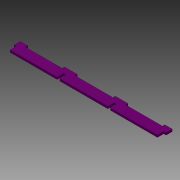
# Autodesk Inventor part: longSlat
Saved by Autodesk Inventor 2015 SP1 (Build 190203100, 203)
## iProperties
Created: 2015-04-09
Part Number: longSlat
Material: Generic
Document SubType Name: Modeling
Designer: Iain
Density: 1 g/cm^3
Appearance: Smooth - Purple
Author: Iain
Autodesk Inventor part; units mm, degrees
ref_plane "YZ Plane" through (0, 0, 0) normal (1, 0, 0) x (0, 1, 0)
sketch "Sketch1" plane through (0, 0, 0) normal (0, 0, 1) x (1, 0, 0)
  line L0 (-590, 40) -> (590, 40)
  line L1 (590, 40) -> (590, -40)
  line L2 (590, -40) -> (-590, -40)
  line L3 (-590, -40) -> (-590, 40)
  point P0 (0, 0)
  point P1 (-590, 0)
  point P2 (0, 40)
  dimension "d0" = 80
  dimension "d1" = 1180
  constraints: 8 end point, 2 midpoint, 2 parallel, 1 horizontal, 1 horizontal alignment, 1 perpendicular, 1 vertical alignment
  measures "d0" distance of L2.end L0.start
  measures "d1" distance of L0.start L0.end
extrude "Extrusion1" add sketch "Sketch1" along normal blind 18
sketch "Sketch2" plane through (0, 0, 18) normal (0, 0, 1) x (1, 0, 0)
  line L0 (590, 40) -> (-590, 40) projected
  line L1 (-590, 40) -> (-590, -40) projected
  line L2 (-590, -40) -> (590, -40) projected
  line L3 (590, -40) -> (590, 40) projected
  line L4 (-590, 58) -> (-531, 58)
  line L5 (-531, 58) -> (-531, 40)
  line L6 (-531, 40) -> (-590, 40)
  line L7 (-590, 40) -> (-590, 58)
  point P0 (0, 0)
  point P1 (-560.5, 40)
  point P2 (0, 40)
  point P3 (-590, 49)
  point P4 (-590, 0)
  dimension "d4" = 18
  dimension "d5" = 59
  constraints: 8 end point, 4 midpoint, 2 parallel, 1 horizontal, 1 horizontal alignment, 1 perpendicular, 1 vertical alignment
  measures "d4" distance of L4.end L5.end
  measures "d5" distance of L4.start L4.end
extrude "Extrusion2" add sketch "Sketch2" against normal blind 18 contours L0 L7 L4 L5
ref_plane "Work Plane1" through (0, -40, 0) normal (-1, 0, 0) x (0, 0, 1)
sketch "Sketch3" plane through (0, 0, 18) normal (0, 0, 1) x (1, 0, 0)
  line L0 (-246.6667, 58) -> (-146.6667, 58)
  line L1 (-146.6667, 58) -> (-146.6667, 40)
  line L2 (-146.6667, 40) -> (-246.6667, 40)
  line L3 (-246.6667, 40) -> (-246.6667, 58)
  line L4 (590, 40) -> (-531, 40) projected
  line L5 (-531, 58) -> (-531, 40) projected
  line L6 (-590, 58) -> (-531, 58) projected
  line L7 (-590, -40) -> (-590, 58) projected
  line L8 (-590, -40) -> (590, -40) projected
  line L9 (590, -40) -> (590, 40) projected
  point P0 (0, 0)
  point P1 (-196.6667, 40)
  point P2 (29.5, 40)
  dimension "d8" = 18
  dimension "d9" = 100
  dimension "d10" = 393.3333
  constraints: 8 end point, 2 midpoint, 2 parallel, 1 horizontal, 1 horizontal alignment, 1 perpendicular
  measures "d8" distance of L0.end L1.end
  measures "d9" distance of L0.start L0.end
  measures "d10" distance from line of L7 point (-196.667, 40)
extrude "Extrusion3" add sketch "Sketch3" against normal blind 18 contours L0 L1 L2 L3
mirror "Mirror1" about plane through (0, -40, 0) normal (-1, 0, 0) of "Extrusion2", "Extrusion3"
sketch "Sketch4" plane through (0, 0, 18) normal (0, 0, 1) x (1, 0, 0)
  line L0 (531, 40) -> (246.6667, 40) projected
  line L1 (246.6667, 40) -> (246.6667, 58) projected
  line L2 (246.6667, 58) -> (146.6667, 58) projected
  line L3 (146.6667, 58) -> (146.6667, 40) projected
  line L4 (146.6667, 40) -> (-146.6667, 40) projected
  line L5 (-146.6667, 58) -> (-146.6667, 40) projected
  line L6 (-246.6667, 58) -> (-146.6667, 58) projected
  line L7 (-246.6667, 40) -> (-246.6667, 58) projected
  line L8 (-246.6667, 40) -> (-531, 40) projected
  line L9 (-531, 58) -> (-531, 40) projected
  line L10 (-590, 58) -> (-531, 58) projected
  line L11 (-590, -40) -> (-590, 58) projected
  line L12 (-590, -40) -> (590, -40) projected
  line L13 (590, -40) -> (590, 58) projected
  line L14 (590, 58) -> (531, 58) projected
  line L15 (531, 58) -> (531, 40) projected
  line L16 (-590, 9) -> (-572, 9)
  line L17 (-572, 9) -> (-572, -40)
  line L18 (-572, -40) -> (-590, -40)
  line L19 (-590, -40) -> (-590, 9)
  point P0 (0, 0)
  point P1 (-590, -15.5)
  point P2 (-590, 9)
  point P3 (-581, -40)
  point P4 (0, -40)
  dimension "d13" = 18
  dimension "d14" = 49
  constraints: 8 end point, 4 midpoint, 2 parallel, 1 horizontal, 1 horizontal alignment, 1 perpendicular, 1 vertical alignment
  measures "d13" distance of L16.start L16.end
  measures "d14" distance of L16.end L17.end
extrude "Extrusion4" cut sketch "Sketch4" against normal blind 18 contours L12 L11 L16 L17
mirror "Mirror2" about plane through (0, -40, 0) normal (-1, 0, 0) of "Extrusion4"
sketch "Sketch5" plane through (0, 0, 18) normal (0, 0, 1) x (1, 0, 0)
  line L0 (-205.6667, 9) -> (-187.6667, 9)
  line L1 (-187.6667, 9) -> (-187.6667, -40)
  line L2 (-187.6667, -40) -> (-205.6667, -40)
  line L3 (-205.6667, -40) -> (-205.6667, 9)
  line L4 (572, -40) -> (572, 9) projected
  line L5 (572, 9) -> (590, 9) projected
  line L6 (590, 9) -> (590, 58) projected
  line L7 (590, 58) -> (531, 58) projected
  line L8 (531, 58) -> (531, 40) projected
  line L9 (531, 40) -> (246.6667, 40) projected
  line L10 (246.6667, 40) -> (246.6667, 58) projected
  line L11 (246.6667, 58) -> (146.6667, 58) projected
  line L12 (146.6667, 58) -> (146.6667, 40) projected
  line L13 (146.6667, 40) -> (-146.6667, 40) projected
  line L14 (-146.6667, 58) -> (-146.6667, 40) projected
  line L15 (-246.6667, 58) -> (-146.6667, 58) projected
  line L16 (-246.6667, 40) -> (-246.6667, 58) projected
  line L17 (-246.6667, 40) -> (-531, 40) projected
  line L18 (-531, 58) -> (-531, 40) projected
  line L19 (-590, 58) -> (-531, 58) projected
  line L20 (-590, 9) -> (-590, 58) projected
  line L21 (-590, 9) -> (-572, 9) projected
  line L22 (-572, 9) -> (-572, -40) projected
  line L23 (-572, -40) -> (572, -40) projected
  point P0 (0, 0)
  point P1 (-196.6667, -40)
  point P2 (0, -40)
  point P3 (-196.6667, 9)
  point P4 (-196.6667, 58)
  dimension "d17" = 18
  dimension "d18" = 49
  constraints: 8 end point, 4 midpoint, 2 parallel, 1 horizontal, 1 horizontal alignment, 1 perpendicular, 1 vertical alignment
  measures "d17" distance of L0.start L0.end
  measures "d18" distance of L0.end L1.end
extrude "Extrusion5" cut sketch "Sketch5" against normal blind 18 contours L0 L1 L2 L3
mirror "Mirror3" about plane through (0, -40, 0) normal (-1, 0, 0) of "Extrusion5"
sketch "Sketch6" plane through (0, 0, 18) normal (0, 0, 1) x (1, 0, 0)
  line L0 (187.6667, -40) -> (187.6667, 9) projected
  line L1 (187.6667, 9) -> (205.6667, 9) projected
  line L2 (205.6667, 9) -> (205.6667, -40) projected
  line L3 (205.6667, -40) -> (572, -40) projected
  line L4 (572, -40) -> (572, 9) projected
  line L5 (572, 9) -> (590, 9) projected
  line L6 (590, 9) -> (590, 58) projected
  line L7 (590, 58) -> (531, 58) projected
  line L8 (531, 58) -> (531, 40) projected
  line L9 (531, 40) -> (246.6667, 40) projected
  line L10 (246.6667, 40) -> (246.6667, 58) projected
  line L11 (246.6667, 58) -> (146.6667, 58) projected
  line L12 (146.6667, 58) -> (146.6667, 40) projected
  line L13 (146.6667, 40) -> (-146.6667, 40) projected
  line L14 (-146.6667, 58) -> (-146.6667, 40) projected
  line L15 (-246.6667, 58) -> (-146.6667, 58) projected
  line L16 (-246.6667, 40) -> (-246.6667, 58) projected
  line L17 (-246.6667, 40) -> (-531, 40) projected
  line L18 (-531, 58) -> (-531, 40) projected
  line L19 (-590, 58) -> (-531, 58) projected
  line L20 (-590, 9) -> (-590, 58) projected
  line L21 (-590, 9) -> (-572, 9) projected
  line L22 (-572, 9) -> (-572, -40) projected
  line L23 (-572, -40) -> (-205.6667, -40) projected
  line L24 (-205.6667, -40) -> (-205.6667, 9) projected
  line L25 (-205.6667, 9) -> (-187.6667, 9) projected
  line L26 (-187.6667, 9) -> (-187.6667, -40) projected
  line L27 (-187.6667, -40) -> (187.6667, -40) projected
  point P0 (0, 0)
  point P1 (-527.825, 40)
  point P2 (-572, 5.825)
  dimension "d21" = 3.175
  dimension "d22" = 3.175
  constraints: 1 horizontal alignment, 1 vertical alignment
  measures "d21" distance from line of L18 point (-527.825, 40)
  measures "d22" distance from line of L21 point (-572, 5.825)
hole "Hole1" at (-527.825, 40, 18) at (-572, 5.825, 18) direction (0, 0, -1) diameter 6.35 end through all
mirror "Mirror4" about plane through (0, -40, 0) normal (-1, 0, 0) of "Hole1"
sketch "Sketch7" plane through (0, 0, 18) normal (0, 0, 1) x (1, 0, 0)
  arc A0 (524.65, 40) -> (531, 40) centre (527.825, 40) ccw projected
  line L0 (524.65, 40) -> (246.6667, 40) projected
  line L1 (246.6667, 40) -> (246.6667, 58) projected
  line L2 (246.6667, 58) -> (146.6667, 58) projected
  line L3 (146.6667, 58) -> (146.6667, 40) projected
  line L4 (146.6667, 40) -> (-146.6667, 40) projected
  line L5 (-146.6667, 58) -> (-146.6667, 40) projected
  line L6 (-246.6667, 58) -> (-146.6667, 58) projected
  line L7 (-246.6667, 40) -> (-246.6667, 58) projected
  line L8 (-246.6667, 40) -> (-524.65, 40) projected
  arc A1 (-531, 40) -> (-524.65, 40) centre (-527.825, 40) ccw projected
  line L9 (-531, 58) -> (-531, 40) projected
  line L10 (-590, 58) -> (-531, 58) projected
  line L11 (-590, 9) -> (-590, 58) projected
  line L12 (-590, 9) -> (-572, 9) projected
  arc A2 (-572, 2.65) -> (-572, 9) centre (-572, 5.825) ccw projected
  line L13 (-572, 2.65) -> (-572, -40) projected
  line L14 (-572, -40) -> (-205.6667, -40) projected
  line L15 (-205.6667, -40) -> (-205.6667, 9) projected
  line L16 (-205.6667, 9) -> (-187.6667, 9) projected
  line L17 (-187.6667, 9) -> (-187.6667, -40) projected
  line L18 (-187.6667, -40) -> (187.6667, -40) projected
  line L19 (187.6667, -40) -> (187.6667, 9) projected
  line L20 (187.6667, 9) -> (205.6667, 9) projected
  line L21 (205.6667, 9) -> (205.6667, -40) projected
  line L22 (205.6667, -40) -> (572, -40) projected
  line L23 (572, -40) -> (572, 2.65) projected
  arc A3 (572, 9) -> (572, 2.65) centre (572, 5.825) ccw projected
  line L24 (572, 9) -> (590, 9) projected
  line L25 (590, 9) -> (590, 58) projected
  line L26 (590, 58) -> (531, 58) projected
  line L27 (531, 58) -> (531, 40) projected
  point P0 (0, 0)
  point P1 (-249.8417, 40)
  point P2 (-205.6667, 5.825)
  dimension "d30" = 3.175
  dimension "d31" = 3.175
  constraints: 1 horizontal alignment, 1 vertical alignment
  measures "d30" distance from line of L7 point (-249.842, 40)
  measures "d31" distance from line of L16 point (-205.667, 5.825)
hole "Hole2" at (-249.8417, 40, 18) at (-205.6667, 5.825, 18) direction (0, 0, -1) diameter 6.35 end through all
ref_plane "Work Plane2" through (-196.6667, -40, 18) normal (1, 0, 0) x (0, 0, -1)
mirror "Mirror5" about plane through (-196.6667, -40, 18) normal (1, 0, 0) of "Hole2"
mirror "Mirror6" about plane through (0, -40, 0) normal (-1, 0, 0) of "Hole2", "Mirror5"
fillet "Fillet1" radius 3.175 4 edges at (-205.6667, -40, 9) (-187.6667, -40, 9) (187.6667, -40, 9) (205.6667, -40, 9)
equation "\"d0\" = legTopDepth"
equation "\"d1\" = tableLength"
equation "\"d2\" = plyThickness"
equation "\"d4\" = legTopTabHeight"
equation "\"d5\" = 0.5 * plyThickness + 0.5 * legTabTotalWidth"
equation "\"d6\" = plyThickness"
equation "\"d8\" = legTopTabHeight"
equation "\"d9\" = legTabTotalWidth"
equation "\"d10\" = 0.333333 * tableLength"
equation "\"d11\" = plyThickness"
equation "\"d13\" = plyThickness"
equation "\"d14\" = legTopSlotDepth"
equation "\"d15\" = plyThickness"
equation "\"d17\" = plyThickness"
equation "\"d18\" = legTopSlotDepth"
equation "\"d19\" = plyThickness"
equation "\"d21\" = 0.5 * millDiameter"
equation "\"d22\" = 0.5 * millDiameter"
equation "\"d23\" = millDiameter"
equation "\"d30\" = 0.5 * millDiameter"
equation "\"d31\" = 0.5 * millDiameter"
equation "\"d32\" = millDiameter"
equation "\"d39\" = 0.5 * millDiameter"
equation "\"plyThickness\" = 18"
equation "\"legHeight\" = 702"
equation "\"tableLength\" = 1180"
equation "\"legTopDepth\" = 80"
equation "\"millDiameter\" = 6.35"
equation "\"legTopTabHeight\" = 18"
equation "\"legTabTotalWidth\" = 100"
equation "\"legTopSlotDepth\" = 49"
body "Solid1"
